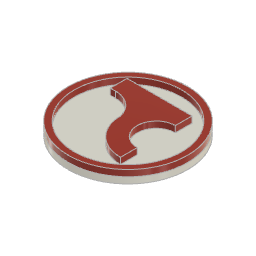
_T With Curve.b8c47f08-3e1f-4f20-9cb6-32d9df6cd3aa (Autodesk Fusion 360 design; units mm, degrees)
Autodesk Fusion 360 part; units mm, degrees
sketch "Sketch1" plane through (0, 0, 0) normal (0, 0, 1) x (1, 0, 0)
  circle A0 centre (0, 0) radius 15.875
  circle A1 centre (0, 0) radius 14.2875
  circle A2 centre (7.3974, 0.1299) radius 9.525
  circle A3 centre (7.3974, 0.1299) radius 5.08
  line L0 (7.3974, 0.1299) -> (7.3974, 9.6549)
  line L1 (7.3974, 0.1299) -> (7.3974, -9.3951)
  line L2 (7.3974, -9.3951) -> (7.3974, -4.9501)
  line L3 (7.3974, -4.9501) -> (-9.906, -4.9501)
  line L4 (-9.906, -4.9501) -> (-9.906, -9.3951)
  line L5 (-9.906, -9.3951) -> (7.3974, -9.3951)
  line L6 (7.3974, 0.1299) -> (-2.1276, 0.1299)
  arc A4 (-8.554, -4.9501) -> (-2.1276, 0.1299) centre (-8.554, 1.6547) ccw
  line L7 (-9.906, 9.6549) -> (7.3974, 9.6549)
  line L8 (7.3974, 5.2099) -> (-9.906, 5.2099)
  line L9 (7.3974, 0.1299) -> (7.3974, 9.6549)
  arc A5 (-2.1276, 0.1299) -> (-8.554, 5.2099) centre (-8.554, -1.3948) ccw
  line L10 (-9.906, 5.2099) -> (-9.906, 9.6549)
  dimension "d16" = 19.05
  dimension "d17" = 10.16
  constraint coincident A0.centre A1.centre
  constraint concentric A2 A3
  constraint coincident A2.centre A3.centre
  constraint coincident A2 L0.end
  constraint vertical L0
  constraint coincident A2 L1.end
  constraint parallel L0 L1
  constraint perpendicular L2 L3
  constraint parallel L2 L4
  constraint parallel L3 L5
  constraint coincident A3 L2.end
  constraint coincident L1 L2.end
  constraint coincident A2 L6.end
  constraint perpendicular L0 L6
  constraint tangent L3 A4
  constraint coincident L3 A4.start
  constraint symmetric A2.centre L6 A3.centre
  constraint symmetric L1.end L6 L0.end
  constraint symmetric L2.end L6 L8.start
  constraint symmetric L3.end L6 L8.end
  constraint symmetric L4.end L6 L7.start
  constraint symmetric A4.end L6 A5.start
  constraint symmetric L6 A4.start A5.end
  constraint symmetric L6 A4 A5
  measures "d16" diameter of A2
  measures "d17" diameter of A3
extrude "Extrude1" add sketch "Sketch1" against normal blind 1 contours A0 A1 A2 | A0 A1 A2 | A1 A2 L3 L4 L5 A4 L7 L8 A5 L10 | A1 A2 A3 L0 L1 L2 L9 | A2 L0 L8 L9 | A2 L7 L8 L10 | A2 L3 L4 L5 | A2 L1 L2 L3 | A2 A3 L6 L8 | A2 L8 A5 | A3 L0 L6 L9 | A3 L0 L1 L9 | A2 L3 A4 | A2 A3 L3 L6 | A3 L1 L6 makes body 1 in component "Base"
extrude "Extrude1'" add sketch "Sketch1" along normal blind 1 separate body contours A0 A1 A2 | A0 A1 A2 | A2 L0 L8 L9 | A2 L7 L8 L10 | A2 L1 L2 L3 | A2 A3 L6 L8 | A2 L8 A5 | A2 A3 L3 L6 makes body 2 at (15.2335, -1.4985, 0) makes body 3 at (-2.738, 7.958, 0) in component "Top"
scale "Scale1" factors (0.6, 0.6, 1) about (-2.1276, 0.1299, 0) bodies 3 2 in component "Top"
scale "Scale1'" factors (0.6, 0.6, 1) about (-2.1276, 0.1299, 0) bodies 1 in component "Base"
component "Base" placed x (1, 0, 0) y (0, 1, 0) z (0, 0, 1) at (0, 0, 0)
component "Top" placed x (1, 0, 0) y (0, 1, 0) z (0, 0, 1) at (0, 0, 0)
